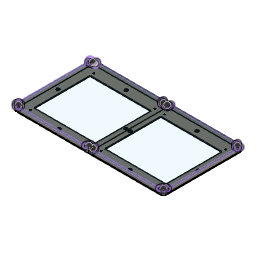
v1.1 (Autodesk Fusion 360 design; units mm, degrees)
Autodesk Fusion 360 part; units mm, degrees
sketch "Sketch1" plane through (0, 0, 0) normal (0, 0, 1) x (1, 0, 0)
  line L0 (192.1478, -6) -> (205.1478, -6) construction
  line L1 (192.1478, -6) -> (179.1478, -6) construction
  circle A0 centre (179.1461, -187.9671) radius 2
  circle A1 centre (13.1478, -188) radius 2
  line L2 (13.1478, -6) -> (13.1478, -16) construction
  circle A2 centre (205.1478, -16) radius 2
  line L3 (13.1478, -198) -> (13.1478, -188) construction
  line L4 (384.1478, -198) -> (371.1478, -198) construction
  line L5 (179.1478, -26) -> (13.1478, -26)
  line L6 (192.1478, -197.9671) -> (179.1478, -197.9671) construction
  line L7 (384.1478, -6) -> (371.1478, -6) construction
  line L8 (179.1478, -6) -> (179.1478, -26) construction
  line L9 (192.1478, -197.9671) -> (0.1478, -198)
  line L10 (205.1478, -197.9671) -> (205.1478, -187.9671) construction
  line L11 (0.1478, -198) -> (0.1478, -6)
  circle A3 centre (179.1478, -16) radius 2
  line L12 (384.1478, -198) -> (384.1478, -6)
  line L13 (371.1478, -26) -> (205.1478, -26)
  line L14 (371.1478, -198) -> (371.1478, -188) construction
  line L15 (205.1478, -26) -> (205.1478, -177.9671)
  line L16 (13.1478, -178) -> (179.1478, -178)
  line L17 (0.1478, -198) -> (13.1478, -198) construction
  line L18 (205.1478, -197.9671) -> (205.1478, -177.9671) construction
  circle A4 centre (205.1478, -187.9671) radius 2
  line L19 (0.1478, -198) -> (13.1478, -198) construction
  line L20 (371.1478, -6) -> (371.1478, -16) construction
  line L21 (192.1478, -6) -> (179.1478, -6) construction
  circle A5 centre (13.1478, -16) radius 2
  circle A6 centre (371.1478, -16) radius 2
  line L22 (192.1478, -6) -> (192.1478, -197.9671) construction
  line L23 (179.1478, -6) -> (179.1478, -16) construction
  line L24 (371.1478, -6) -> (371.1478, -26) construction
  line L25 (205.1478, -6) -> (205.1478, -16) construction
  line L26 (13.1478, -26) -> (13.1478, -178)
  line L27 (384.1478, -6) -> (0.1478, -6)
  line L28 (179.1478, -197.9671) -> (179.1461, -187.9671) construction
  line L29 (13.1478, -198) -> (13.1478, -178) construction
  line L30 (0.1478, -6) -> (13.1478, -6) construction
  line L31 (179.1478, -178) -> (179.1478, -26)
  line L32 (192.1478, -197.9671) -> (205.1478, -197.9671) construction
  line L33 (0.1478, -6) -> (0.1478, -198)
  line L34 (205.1478, -177.9671) -> (371.1478, -177.9671)
  circle A7 centre (371.1478, -188) radius 2
  line L35 (384.1478, -6) -> (371.1478, -6) construction
  line L36 (371.1478, -177.9671) -> (371.1478, -26)
  line L37 (0.1478, -198) -> (384.1478, -198)
  line L38 (192.1478, -197.9671) -> (205.1478, -197.9671) construction
  line L39 (384.1478, -6) -> (384.1478, 12.0213) construction
  line L40 (0.1478, -6) -> (-9.0446, 3.1924) construction
  line L41 (0.1478, -6) -> (15, -6) construction
  circle A8 centre (-4.4484, -1.4038) radius 6.5
  line L42 (0.1478, -198) -> (-9.0446, -207.1924) construction
  line L43 (384.1478, -198) -> (393.3402, -207.1924) construction
  line L44 (384.1478, -198) -> (399, -198) construction
  line L45 (384.1478, -6) -> (393.3402, 3.1924) construction
  line L46 (384.1478, -6) -> (399, -6) construction
  circle A9 centre (388.744, -1.4038) radius 6.5
  circle A10 centre (388.744, -202.5962) radius 6.5
  circle A11 centre (-4.4484, -202.5962) radius 6.5
  line L47 (-10.9305, -1.8855) -> (-10.9484, -202.5956)
  line L48 (-4.4484, -209.0962) -> (388.744, -209.0962)
  line L49 (395.244, -202.5962) -> (395.244, -1.4038)
  line L50 (-4.4484, 5.0962) -> (388.744, 5.0962)
  line L51 (388.744, -202.5962) -> (395.244, -202.5962) construction
  line L52 (-4.4484, -1.4038) -> (-4.4484, 5.0962) construction
  point P0 (13, -13)
  dimension "d13" = 192
  dimension "d14" = 192
  dimension "d15" = 384
  dimension "d16" = 384
  dimension "d20" = 13
  dimension "d21" = 10
  dimension "d22" = 4
  dimension "d23" = 13
  dimension "d24" = 10
  dimension "d25" = 13
  dimension "d26" = 10
  dimension "d27" = 13
  dimension "d28" = 10
  dimension "d29" = 13
  dimension "d30" = 10
  dimension "d31" = 13
  dimension "d32" = 10
  dimension "d33" = 13
  dimension "d34" = 10
  dimension "d35" = 13
  dimension "d36" = 10
  dimension "d37" = 4
  dimension "d38" = 4
  dimension "d39" = 4
  dimension "d40" = 4
  dimension "d41" = 4
  dimension "d42" = 4
  dimension "d43" = 4
  dimension "d44" = 13
  dimension "d45" = 20
  dimension "d46" = 13
  dimension "d47" = 20
  dimension "d48" = 13
  dimension "d49" = 20
  dimension "d50" = 13
  dimension "d51" = 20
  dimension "d69" = 135
  dimension "d70" = 13
  dimension "d71" = 13
  dimension "d72" = 45
  dimension "d73" = 13
  dimension "d74" = 13
  dimension "d75" = 45
  dimension "d104" = 135
  constraint perpendicular L11 L30
  constraint perpendicular L2 L30
  constraint coincident L2.end A5.centre
  constraint perpendicular L7 L12
  constraint perpendicular L7 L20
  constraint perpendicular L4 L12
  constraint perpendicular L14 L37
  constraint perpendicular L19 L33
  constraint perpendicular L3 L19
  constraint midpoint L0.start L27
  constraint perpendicular L22 L37
  constraint perpendicular L6 L22
  constraint perpendicular L9 L28
  constraint perpendicular L21 L22
  constraint perpendicular L21 L23
  constraint perpendicular L0 L22
  constraint perpendicular L25 L27
  constraint perpendicular L22 L32
  constraint perpendicular L10 L32
  constraint coincident A1.centre L3.end
  constraint coincident A3.centre L23.end
  constraint coincident A0.centre L28.end
  constraint coincident A2.centre L25.end
  constraint coincident L10.end A4.centre
  constraint coincident L14.end A7.centre
  constraint coincident L20.end A6.centre
  constraint perpendicular L11 L17
  constraint perpendicular L17 L29
  constraint perpendicular L1 L22
  constraint perpendicular L1 L8
  constraint horizontal L16
  constraint vertical L31
  constraint horizontal L5
  constraint vertical L26
  constraint perpendicular L22 L38
  constraint perpendicular L18 L38
  constraint perpendicular L20 L35
  constraint perpendicular L24 L35
  constraint horizontal L34
  constraint vertical L36
  constraint horizontal L13
  constraint vertical L15
  constraint perpendicular L7 L39
  constraint horizontal L41
  constraint coincident L40.end A8
  constraint coincident L11.end A8
  constraint horizontal L44
  constraint horizontal L46
  constraint coincident L45.end A9
  constraint coincident L7.start A9
  constraint coincident L43.end A10
  constraint coincident L4.start A10
  constraint coincident L42.end A11
  constraint coincident L9.end A11
  constraint coincident A8 L47.start
  constraint coincident A11 L47.end
  constraint tangent A11 L47
  constraint coincident A10 L48.end
  constraint tangent A10 L48
  constraint coincident A9 L49.end
  constraint tangent A9 L49
  constraint perpendicular L46 L49
  constraint coincident A9 L50.end
  constraint tangent A9 L50
  constraint perpendicular L49 L50
  constraint coincident L42 A11.centre
  constraint coincident L43 A10.centre
  constraint coincident L45 A9.centre
  constraint coincident L40 A8.centre
  constraint coincident A11 L48.start
  constraint tangent A11 L48
  constraint coincident A10.centre L51.start
  constraint coincident A10 L49.start
  constraint parallel L48 L51
  constraint coincident L49.start L51.end
  constraint coincident A8.centre L52.start
  constraint coincident A8 L50.start
  constraint vertical L52
  constraint coincident L50.start L52.end
  measures "d13" distance of L11.end L9.end
  measures "d14" distance of L4.start L7.start
  measures "d15" distance of L7.start L11.end
  measures "d16" distance of L4.start L9.end
  measures "d20" distance of L2.start L11.end
  measures "d21" distance of L2.start L2.end
  measures "d22" diameter of A5
  measures "d23" distance of L7.end L7.start
  measures "d24" distance of L7.end L20.end
  measures "d25" distance of L4.end L4.start
  measures "d26" distance of L4.end L14.end
  measures "d27" distance of L3.start L9.end
  measures "d28" distance of L3.start A1.centre
  measures "d29" distance of L6.end L6.start
  measures "d30" distance of L6.end A0.centre
  measures "d31" distance of L0.start L1.end
  measures "d32" distance of A3.centre L1.end
  measures "d33" distance of L0.start L0.end
  measures "d34" distance of A2.centre L0.end
  measures "d35" distance of L10.start L6.start
  measures "d36" distance of L10.end L10.start
  measures "d37" diameter of A1
  measures "d38" diameter of A3
  measures "d39" diameter of A0
  measures "d40" diameter of A2
  measures "d41" diameter of A4
  measures "d42" diameter of A7
  measures "d43" diameter of A6
  measures "d44" distance of L9.end L3.start
  measures "d45" distance of L16.start L3.start
  measures "d46" distance of L0.start L1.end
  measures "d47" distance of L5.start L1.end
  measures "d48" distance of L6.start L10.start
  measures "d49" distance of L10.start L15.end
  measures "d50" distance of L7.start L7.end
  measures "d51" distance of L13.start L7.end
  measures "d69" angle of L40 L41
  measures "d70" distance of L11.end L40.end
  measures "d71" distance of L9.end L42.end
  measures "d72" angle of L43 L44
  measures "d73" distance of L4.start L43.end
  measures "d74" distance of L7.start L45.end
  measures "d75" angle of L45 L46
  measures "d104" angle of L37 L42
extrude "Extrude1" add sketch "Sketch1" along normal blind 2 makes body 1
sketch "Sketch3" plane through (0, 0, 2) normal (0, 0, 1) x (-1, 0, 0)
  arc A0 (-395.244, 1.4038) -> (-388.744, -5.0962) centre (-388.744, 1.4038) ccw
  line L0 (-388.744, -5.0962) -> (4.4484, -5.0962)
  arc A1 (4.4484, -5.0962) -> (10.9305, 1.8855) centre (4.4484, 1.4038) ccw
  circle A2 centre (4.4484, 1.4038) radius 5.5
  circle A3 centre (4.4484, 202.5962) radius 5.5
  circle A4 centre (-388.744, 202.5962) radius 5.5
  circle A5 centre (-388.744, 1.4038) radius 5.5
  line L1 (-388.744, -4.0962) -> (4.4484, -4.0962)
  line L2 (9.9484, 1.4038) -> (9.9484, 202.5962)
  line L3 (3.3138, 207.9779) -> (-388.7423, 208.0962)
  line L4 (-394.244, 202.5962) -> (-394.244, 1.4038)
  line L5 (-192.1478, -4.0962) -> (-192.7143, 208.037) construction
  circle A6 centre (-187.1611, 0.9038) radius 5
  circle A7 centre (-197.1612, 0.9038) radius 5
  circle A8 centre (-187.7009, 203.0355) radius 5
  circle A9 centre (-197.701, 203.0385) radius 5
  line L6 (-182.7009, 203.0355) -> (-182.7009, 208.034)
  line L7 (-202.7008, 203.0726) -> (-202.667, 208.04)
  line L8 (-187.1611, 5.9038) -> (-197.1612, 5.9038)
  line L9 (-202.1612, 0.9038) -> (-202.1612, -4.0962)
  line L10 (-182.1611, 0.9038) -> (-182.1611, -4.0962)
  line L11 (-383.662, 197.9997) -> (-384, 6)
  line L12 (0.338, 197.9997) -> (-383.662, 197.9997)
  line L13 (0, 6) -> (0.338, 197.9997)
  line L14 (-384, 6) -> (0, 6)
  line L15 (4.4484, 6.9038) -> (9.9484, 6.9038)
  line L16 (-1.0516, 1.4038) -> (-1.0516, -4.0962)
  line L17 (-383.244, 1.4038) -> (-383.244, -4.0962)
  line L18 (-388.744, 6.9038) -> (-394.244, 6.9038)
  line L19 (-388.744, 197.0962) -> (-394.244, 197.0962)
  line L20 (-383.244, 202.5962) -> (-383.244, 208.0945)
  line L21 (4.4484, 197.0962) -> (9.9484, 197.0962)
  line L22 (-1.0516, 202.5962) -> (-1.0516, 207.9792)
  circle A10 centre (-13.1478, 188) radius 2
  circle A11 centre (-179.1461, 187.9671) radius 2
  circle A12 centre (-205.1478, 16) radius 2
  circle A13 centre (-179.1478, 16) radius 2
  circle A14 centre (-205.1478, 187.9671) radius 2
  circle A15 centre (-13.1478, 16) radius 2
  circle A16 centre (-371.1478, 16) radius 2
  line L23 (-179.1478, 26) -> (-179.1478, 178)
  line L24 (-179.1478, 178) -> (-13.1478, 178)
  line L25 (-13.1478, 178) -> (-13.1478, 26)
  line L26 (-13.1478, 26) -> (-179.1478, 26)
  line L27 (-371.1478, 26) -> (-371.1478, 177.9671)
  line L28 (-371.1478, 177.9671) -> (-205.1478, 177.9671)
  line L29 (-205.1478, 177.9671) -> (-205.1478, 26)
  line L30 (-205.1478, 26) -> (-371.1478, 26)
  circle A17 centre (-371.1478, 188) radius 2
  line L31 (10.9305, 1.8855) -> (10.9484, 202.5956)
  arc A18 (10.9484, 202.5956) -> (4.4484, 209.0962) centre (4.4484, 202.5962) ccw
  line L32 (4.4484, 209.0962) -> (-388.744, 209.0962)
  arc A19 (-388.744, 209.0962) -> (-395.244, 202.5962) centre (-388.744, 202.5962) ccw
  line L33 (-395.244, 202.5962) -> (-395.244, 1.4038)
  line L34 (-187.7009, 198.0355) -> (-197.7025, 198.0385)
  dimension "d76" = 11
  dimension "d77" = 11
  dimension "d78" = 11
  dimension "d79" = 11
  dimension "d80" = 5
  dimension "d81" = 5
  dimension "d82" = 5
  dimension "d83" = 5
  dimension "d85" = 192
  dimension "d87" = 384
  constraint concentric A1 A2
  constraint concentric A0 A5
  constraint coincident A5 L1.start
  constraint coincident A2 L1.end
  constraint tangent A2 L1
  constraint parallel L0 L1
  constraint coincident A2 L2.start
  constraint coincident A3 L2.end
  constraint tangent A3 L2
  constraint coincident A3 L3.start
  constraint coincident A4 L3.end
  constraint tangent A4 L3
  constraint coincident A4 L4.start
  constraint coincident A5 L4.end
  constraint tangent A5 L4
  constraint midpoint L1 L5.start
  constraint midpoint L3 L5.end
  constraint tangent L1 A6
  constraint tangent L5 A6
  constraint tangent L5 A7
  constraint tangent L1 A7
  constraint tangent L5 A8
  constraint tangent L3 A8
  constraint tangent L5 A9
  constraint tangent L3 A9
  constraint coincident A8 L6.start
  constraint coincident L3 L6.end
  constraint tangent A8 L6
  constraint vertical L6
  constraint coincident A9 L7.start
  constraint coincident L3 L7.end
  constraint tangent A9 L7
  constraint coincident A6 L8.start
  constraint coincident A7 L8.end
  constraint tangent A7 L8
  constraint horizontal L8
  constraint coincident A7 L9.start
  constraint coincident L1 L9.end
  constraint tangent A7 L9
  constraint perpendicular L1 L9
  constraint coincident A6 L10.start
  constraint coincident L1 L10.end
  constraint tangent A6 L10
  constraint perpendicular L1 L10
  constraint coincident A2 L15.start
  constraint coincident L2 L15.end
  constraint tangent A2 L15
  constraint horizontal L15
  constraint coincident A2 L16.start
  constraint coincident L1 L16.end
  constraint tangent A2 L16
  constraint perpendicular L1 L16
  constraint coincident A5 L17.start
  constraint coincident L1 L17.end
  constraint tangent A5 L17
  constraint perpendicular L1 L17
  constraint coincident A5 L18.start
  constraint coincident L4 L18.end
  constraint tangent A5 L18
  constraint perpendicular L4 L18
  constraint coincident A4 L19.start
  constraint coincident L4 L19.end
  constraint tangent A4 L19
  constraint perpendicular L4 L19
  constraint coincident A4 L20.start
  constraint coincident L3 L20.end
  constraint tangent A4 L20
  constraint vertical L20
  constraint coincident A3 L21.start
  constraint coincident L2 L21.end
  constraint tangent A3 L21
  constraint horizontal L21
  constraint coincident A3 L22.start
  constraint coincident L3 L22.end
  constraint tangent A3 L22
  constraint vertical L22
  constraint coincident A3.centre A18.centre
  constraint coincident A4.centre A19.centre
  constraint coincident A8 L34.start
  constraint coincident A9 L34.end
  constraint tangent A9 L34
  measures "d76" diameter of A2
  measures "d77" diameter of A3
  measures "d78" diameter of A4
  measures "d79" diameter of A5
  measures "d80" radius of A6
  measures "d81" radius of A7
  measures "d82" radius of A8
  measures "d83" radius of A9
  measures "d85" distance of L13.start L12.start
  measures "d87" distance of L13.start L11.end
extrude "Extrude3" add sketch "Sketch3" along normal blind 10.5 contours A0 L0 A1 L31 A18 L32 A19 L33 | A2 | A2 L2 L15 | A8 A9 L34 | A2 L1 L16 | A3 L2 L21 | L1 A6 L10 | A3 | L1 A6 A7 | A6 | A3 L3 L22 | L1 A7 L9 | A7 | A6 A7 L8 | L3 A8 L6 | A5 L1 L17 | L3 A8 A9 | A8 | A5 | L3 A9 L7 | A9 | A5 L4 L18 | A4 L3 L20 | A4 L4 L19 | A4 bodies 1
sketch "Sketch4" plane through (0, 0, 12.5) normal (0, 0, 1) x (-1, 0, 0)
  arc A0 (4.4484, -5.0962) -> (10.9305, 1.8855) centre (4.4484, 1.4038) ccw
  line L0 (-388.744, -5.0962) -> (4.4484, -5.0962)
  circle A1 centre (4.4484, 1.4038) radius 5
  circle A2 centre (-187.1611, 0.9038) radius 5
  circle A3 centre (-197.1612, 0.9038) radius 5
  circle A4 centre (-388.744, 1.4038) radius 5
  circle A5 centre (-388.744, 202.5962) radius 5
  circle A6 centre (-197.701, 203.0385) radius 5
  circle A7 centre (-187.7009, 203.0355) radius 5
  circle A8 centre (4.4484, 202.5962) radius 5
  line L1 (10.9305, 1.8855) -> (10.9484, 202.5956)
  arc A9 (10.9484, 202.5956) -> (4.4484, 209.0962) centre (4.4484, 202.5962) ccw
  line L2 (4.4484, 209.0962) -> (-388.744, 209.0962)
  arc A10 (-388.744, 209.0962) -> (-395.244, 202.5962) centre (-388.744, 202.5962) ccw
  line L3 (-395.244, 202.5962) -> (-395.244, 1.4038)
  arc A11 (-395.244, 1.4038) -> (-388.744, -5.0962) centre (-388.744, 1.4038) ccw
  line L4 (-202.1612, -4.0962) -> (-383.244, -4.0962)
  arc A12 (-383.244, 1.4038) -> (-388.744, 6.9038) centre (-388.744, 1.4038) ccw
  line L5 (-394.244, 6.9038) -> (-394.244, 197.0962)
  arc A13 (-388.744, 197.0962) -> (-383.244, 202.5962) centre (-388.744, 202.5962) ccw
  line L6 (-383.244, 208.0945) -> (-202.667, 208.04)
  arc A14 (-1.0516, 202.5962) -> (4.4484, 197.0962) centre (4.4484, 202.5962) ccw
  line L7 (9.9484, 197.0962) -> (9.9484, 6.9038)
  arc A15 (4.4484, 6.9038) -> (-1.0516, 1.4038) centre (4.4484, 1.4038) ccw
  arc A16 (-187.7009, 198.0355) -> (-182.7009, 203.0355) centre (-187.7009, 203.0355) ccw
  line L8 (-182.7009, 203.0355) -> (-182.7009, 208.034)
  line L9 (-182.7009, 208.034) -> (-1.0516, 207.9792)
  line L10 (-1.0516, 207.9792) -> (-1.0516, 202.5962)
  line L11 (4.4484, 197.0962) -> (9.9484, 197.0962)
  line L12 (9.9484, 6.9038) -> (4.4484, 6.9038)
  line L13 (-1.0516, 1.4038) -> (-1.0516, -4.0962)
  line L14 (-1.0516, -4.0962) -> (-182.1611, -4.0962)
  line L15 (-182.1611, -4.0962) -> (-182.1611, 0.9038)
  arc A17 (-182.1611, 0.9038) -> (-187.1611, 5.9038) centre (-187.1611, 0.9038) ccw
  line L16 (-187.1611, 5.9038) -> (-197.1612, 5.9038)
  arc A18 (-197.1612, 5.9038) -> (-202.1612, 0.9038) centre (-197.1612, 0.9038) ccw
  line L17 (-202.1612, 0.9038) -> (-202.1612, -4.0962)
  line L18 (-394.244, 197.0962) -> (-388.744, 197.0962)
  line L19 (-383.244, 202.5962) -> (-383.244, 208.0945)
  line L20 (-202.667, 208.04) -> (-202.7008, 203.0726)
  arc A19 (-202.7008, 203.0726) -> (-197.7025, 198.0385) centre (-197.701, 203.0385) ccw
  line L21 (-197.7025, 198.0385) -> (-187.7009, 198.0355)
  line L22 (-383.244, -4.0962) -> (-383.244, 1.4038)
  line L23 (-388.744, 6.9038) -> (-394.244, 6.9038)
  point P0 (3.9781, 2.1111)
  dimension "d90" = 10
  dimension "d91" = 10
  dimension "d92" = 10
  dimension "d93" = 10
  dimension "d94" = 10
  dimension "d95" = 10
  dimension "d96" = 10
  dimension "d97" = 10
  constraint coincident A2.centre A17.centre
  constraint coincident A3.centre A18.centre
  constraint coincident A5.centre A10.centre
  constraint coincident A4.centre A11.centre
  constraint coincident A6.centre A19.centre
  constraint coincident A7.centre A16.centre
  constraint coincident A8.centre A9.centre
  constraint coincident A0.centre A1.centre
  measures "d90" diameter of A1
  measures "d91" diameter of A2
  measures "d92" diameter of A3
  measures "d93" diameter of A4
  measures "d94" diameter of A5
  measures "d95" diameter of A6
  measures "d96" diameter of A7
  measures "d97" diameter of A8
extrude "Extrude4" cut sketch "Sketch4" against normal blind 3.2 contours A1 | A2 A17 | A3 A18 | A7 A16 | A6 A19 | A4 | A5 | A8 bodies 1
extrude "Extrude5" add 3 faces at (-9.9182, -4.1722, 12.5) (192.3118, -3.3983, 12.5) (192.5511, -200.5431, 12.5) along direction (0, 0, 1) blind 3 separate body on bodies 1 makes body 2
sketch "Sketch7" plane through (0, 0, 15.5) normal (0, 0, 1) x (-1, 0, 0)
  arc A0 (-197.7025, 198.0385) -> (-202.7008, 203.0726) centre (-197.701, 203.0385) ccw
  line L0 (-197.7025, 198.0385) -> (-187.7009, 198.0355)
  arc A1 (-182.7009, 203.0355) -> (-187.7009, 198.0355) centre (-187.7009, 203.0355) ccw
  line L1 (-182.7009, 203.0355) -> (-182.7009, 208.034)
  line L2 (-182.7009, 208.034) -> (-1.0516, 207.9792)
  line L3 (-1.0516, 207.9792) -> (-1.0516, 202.5962)
  arc A2 (-1.0516, 202.5962) -> (4.4484, 197.0962) centre (4.4484, 202.5962) ccw
  line L4 (4.4484, 197.0962) -> (9.9484, 197.0962)
  line L5 (9.9484, 197.0962) -> (9.9484, 6.9038)
  line L6 (9.9484, 6.9038) -> (4.4484, 6.9038)
  arc A3 (4.4484, 6.9038) -> (-1.0516, 1.4038) centre (4.4484, 1.4038) ccw
  line L7 (-1.0516, 1.4038) -> (-1.0516, -4.0962)
  line L8 (-1.0516, -4.0962) -> (-182.1611, -4.0962)
  line L9 (-182.1611, -4.0962) -> (-182.1611, 0.9038)
  arc A4 (-187.1611, 5.9038) -> (-182.1611, 0.9038) centre (-187.1611, 0.9038) ccw
  line L10 (-187.1611, 5.9038) -> (-197.1612, 5.9038)
  arc A5 (-202.1612, 0.9038) -> (-197.1612, 5.9038) centre (-197.1612, 0.9038) ccw
  line L11 (-202.1612, 0.9038) -> (-202.1612, -4.0962)
  line L12 (-202.1612, -4.0962) -> (-383.244, -4.0962)
  line L13 (-383.244, -4.0962) -> (-383.244, 1.4038)
  arc A6 (-383.244, 1.4038) -> (-388.744, 6.9038) centre (-388.744, 1.4038) ccw
  line L14 (-388.744, 6.9038) -> (-394.244, 6.9038)
  line L15 (-394.244, 6.9038) -> (-394.244, 197.0962)
  line L16 (-394.244, 197.0962) -> (-388.744, 197.0962)
  arc A7 (-388.744, 197.0962) -> (-383.244, 202.5962) centre (-388.744, 202.5962) ccw
  line L17 (-383.244, 202.5962) -> (-383.244, 208.0945)
  line L18 (-383.244, 208.0945) -> (-202.667, 208.04)
  line L19 (-202.667, 208.04) -> (-202.7008, 203.0726)
  circle A8 centre (-388.744, 202.5962) radius 5
  circle A9 centre (4.4484, 1.4038) radius 5
  circle A10 centre (-388.744, 1.4038) radius 5
  circle A11 centre (4.4484, 202.5962) radius 5
  line L20 (-395.244, 202.5962) -> (-395.244, 1.4038)
  arc A12 (-395.244, 1.4038) -> (-388.744, -5.0962) centre (-388.744, 1.4038) ccw
  line L21 (-388.744, -5.0962) -> (4.4484, -5.0962)
  arc A13 (4.4484, -5.0962) -> (10.9305, 1.8855) centre (4.4484, 1.4038) ccw
  line L22 (10.9305, 1.8855) -> (10.9484, 202.5956)
  arc A14 (10.9484, 202.5956) -> (4.4484, 209.0962) centre (4.4484, 202.5962) ccw
  line L23 (4.4484, 209.0962) -> (-388.744, 209.0962)
  arc A15 (-388.744, 209.0962) -> (-395.244, 202.5962) centre (-388.744, 202.5962) ccw
  circle A16 centre (4.4484, 202.5962) radius 6.5
  circle A17 centre (4.4484, 1.4038) radius 6.5
  circle A18 centre (-388.744, 1.4038) radius 6.5
  circle A19 centre (-388.744, 202.5962) radius 6.5
  spline S0 degree 5 poles (10.9467, 1.2553) (10.9468, 9.309) (10.9469, 25.4162) (10.9471, 49.577) (10.9474, 81.7915) (10.9477, 122.0595) (10.948, 154.274) (10.9482, 178.4348) (10.9483, 194.542) (10.9484, 202.5956) knots 0 0 0 0 0 0 0.2 0.4 0.6 0.8 1 1 1 1 1 1
  line L24 (4.4484, 209.0962) -> (-388.744, 209.0962)
  line L25 (-395.244, 202.5962) -> (-395.244, 1.4038)
  line L26 (-388.744, -5.0962) -> (4.4484, -5.0962)
  constraint concentric A2 A16
  constraint concentric A3 A17
  constraint concentric A6 A18
  constraint concentric A7 A19
  constraint coincident A13 S0.start
  constraint coincident A17 S0.start
  constraint coincident L22.end A14.start
  constraint coincident A14.end L23.start
  constraint coincident L23.end A15.start
  constraint coincident L20.start A15.end
  constraint coincident L20.end A12.start
  constraint coincident A12.end L21.start
  constraint coincident L21.end A13.start
extrude "Extrude7" add sketch "Sketch7" along normal blind 0.5 contours A4 L10 A5 | A0 A1 L1 L2 L3 L4 L5 L6 L7 L8 L9 A4 A5 L11 L12 L13 L14 L15 L16 L17 L18 L19 A16 A17 A18 A19 | A0 A1 L1 L2 L3 L17 L18 L19 L23 A16 A19 L24 | A0 L0 A1 | L16 A7 L17 A19 | L16 A7 L17 A15 A19 | L3 A2 L4 A14 A16 | L3 A2 L4 A16 | L4 L5 L6 L22 A16 A17 S0 | L14 L15 L16 L20 A18 A19 L25 | L13 A6 L14 A12 A18 | L6 A3 L7 A13 A17 S0 | L7 L8 L9 A4 A5 L11 L12 L13 L21 A17 A18 L26 | L13 A6 L14 A18 | L6 A3 L7 A17 | A8 | A9 | A10 | A11 bodies 2
sketch "Sketch8" plane through (0, 0, 2) normal (0, 0, 1) x (-1, 0, 0)
  line L0 (-197.1612, 5.9038) -> (-187.1611, 5.9038)
  arc A0 (-182.1611, 0.9038) -> (-187.1611, 5.9038) centre (-187.1611, 0.9038) ccw
  line L1 (-182.1611, 0.9038) -> (-182.1611, -4.0962)
  line L2 (-182.1611, -4.0962) -> (-1.0516, -4.0962)
  line L3 (-1.0516, -4.0962) -> (-1.0516, 1.4038)
  arc A1 (4.4484, 6.9038) -> (-1.0516, 1.4038) centre (4.4484, 1.4038) ccw
  line L4 (4.4484, 6.9038) -> (9.9484, 6.9038)
  line L5 (9.9484, 6.9038) -> (9.9484, 197.0962)
  line L6 (9.9484, 197.0962) -> (4.4484, 197.0962)
  arc A2 (-1.0516, 202.5962) -> (4.4484, 197.0962) centre (4.4484, 202.5962) ccw
  line L7 (-1.0516, 202.5962) -> (-1.0516, 207.9792)
  line L8 (-1.0516, 207.9792) -> (-182.7009, 208.034)
  line L9 (-182.7009, 208.034) -> (-182.7009, 203.0355)
  arc A3 (-187.7009, 198.0355) -> (-182.7009, 203.0355) centre (-187.7009, 203.0355) ccw
  line L10 (-187.7009, 198.0355) -> (-197.7025, 198.0385)
  circle A4 centre (-179.1478, 16) radius 2
  circle A5 centre (-13.1478, 16) radius 2
  line L11 (-179.1478, 26) -> (-179.1478, 178)
  line L12 (-179.1478, 178) -> (-13.1478, 178)
  line L13 (-13.1478, 178) -> (-13.1478, 26)
  line L14 (-13.1478, 26) -> (-179.1478, 26)
  circle A6 centre (-13.1478, 188) radius 2
  circle A7 centre (-179.1461, 187.9671) radius 2
  line L15 (-13.1478, 102) -> (-179.1478, 102) construction
  line L16 (-96.1478, 26) -> (-96.1478, 178) construction
  line L17 (-96.1478, 26) -> (-96.1478, -4.0962) construction
  line L18 (-13.1478, 102) -> (9.9484, 102) construction
  line L19 (-179.1478, 102) -> (-179.1526, 101.9998) construction
  line L20 (-179.1526, 101.9998) -> (-194.2518, 101.9998) construction
  line L21 (-96.1478, 178) -> (-96.1388, 208.0079) construction
  circle A8 centre (-96.1478, 10.9519) radius 4
  circle A9 centre (-1.5997, 102) radius 4
  circle A10 centre (-186.7022, 101.9998) radius 4
  circle A11 centre (-96.1433, 193.004) radius 4
  circle A12 centre (-288.1649, 10.9605) radius 4
  circle A13 centre (-382.7049, 102.017) radius 4
  circle A14 centre (-288.1532, 193.0125) radius 4
  circle A15 centre (-198.2326, 101.9709) radius 4
  line L22 (-194.2963, 43.9518) -> (-190.2963, 43.9518)
  line L23 (-190.2963, 43.9518) -> (-190.2963, 63.9518)
  line L24 (-190.2963, 63.9518) -> (-194.2963, 63.9518)
  line L25 (-194.2963, 63.9518) -> (-194.2963, 43.9518)
  line L26 (-194.2963, 43.9518) -> (-190.2963, 63.9518) construction
  line L27 (-190.2963, 43.9518) -> (-194.2963, 63.9518) construction
  line L28 (-190.5666, 160.0184) -> (-194.5666, 160.0184)
  line L29 (-194.5666, 160.0184) -> (-194.5666, 140.0184)
  line L30 (-194.5666, 140.0184) -> (-190.5666, 140.0184)
  line L31 (-190.5666, 140.0184) -> (-190.5666, 160.0184)
  line L32 (-190.5666, 160.0184) -> (-194.5666, 140.0184) construction
  line L33 (-194.5666, 160.0184) -> (-190.5666, 140.0184) construction
  arc A16 (-202.7008, 203.0726) -> (-197.7025, 198.0385) centre (-197.701, 203.0385) ccw
  line L34 (-202.7008, 203.0726) -> (-202.667, 208.04)
  line L35 (-202.667, 208.04) -> (-383.244, 208.0945)
  line L36 (-383.244, 208.0945) -> (-383.244, 202.5962)
  arc A17 (-388.744, 197.0962) -> (-383.244, 202.5962) centre (-388.744, 202.5962) ccw
  line L37 (-388.744, 197.0962) -> (-394.244, 197.0962)
  line L38 (-394.244, 197.0962) -> (-394.244, 6.9038)
  line L39 (-394.244, 6.9038) -> (-388.744, 6.9038)
  arc A18 (-383.244, 1.4038) -> (-388.744, 6.9038) centre (-388.744, 1.4038) ccw
  line L40 (-383.244, 1.4038) -> (-383.244, -4.0962)
  line L41 (-383.244, -4.0962) -> (-202.1612, -4.0962)
  line L42 (-202.1612, -4.0962) -> (-202.1612, 0.9038)
  arc A19 (-197.1612, 5.9038) -> (-202.1612, 0.9038) centre (-197.1612, 0.9038) ccw
  circle A20 centre (-205.1478, 16) radius 2
  circle A21 centre (-205.1478, 187.9671) radius 2
  circle A22 centre (-371.1478, 16) radius 2
  line L43 (-371.1478, 26) -> (-371.1478, 177.9671)
  line L44 (-371.1478, 177.9671) -> (-205.1478, 177.9671)
  line L45 (-205.1478, 177.9671) -> (-205.1478, 26)
  line L46 (-205.1478, 26) -> (-371.1478, 26)
  circle A23 centre (-371.1478, 188) radius 2
  line L47 (-192.7017, 198.037) -> (-192.4315, 101.9998) construction
  line L48 (-192.4315, 101.9998) -> (-192.1612, 5.9038) construction
  line L49 (-179.1526, 101.9998) -> (-190.7022, 101.9926)
  line L50 (-192.4315, 101.9915) -> (-205.1478, 101.9836)
  line L51 (-190.7022, 101.9926) -> (-192.4315, 101.9915)
  point P0 (-192.2963, 53.9518)
  point P1 (-192.5666, 150.0184)
  dimension "d107" = 8
  dimension "d108" = 8
  dimension "d109" = 8
  dimension "d110" = 8
  dimension "d119" = 4
  dimension "d120" = 20
  dimension "d121" = 4
  dimension "d122" = 20
  constraint midpoint L13 L15.start
  constraint midpoint L11 L15.end
  constraint midpoint L14 L16.start
  constraint midpoint L12 L16.end
  constraint coincident L2 L17.end
  constraint perpendicular L2 L17
  constraint midpoint L5 L18.end
  constraint horizontal L20
  constraint coincident L8 L21.end
  constraint perpendicular L8 L21
  constraint midpoint L17 A8.centre
  constraint midpoint L18 A9.centre
  constraint midpoint L20 A10.centre
  constraint midpoint L21 A11.centre
  constraint horizontal L22
  constraint perpendicular L22 L23
  constraint parallel L22 L24
  constraint parallel L23 L25
  constraint coincident L26 P0
  constraint coincident L27 P0
  constraint horizontal L28
  constraint perpendicular L28 L29
  constraint parallel L28 L30
  constraint parallel L29 L31
  constraint coincident L32 P1
  constraint coincident L33 P1
  constraint midpoint L10 L47.start
  constraint midpoint L0 L48.end
  constraint coincident L20 L47.end
  constraint midpoint P0 L48
  constraint midpoint P1 L47
  constraint midpoint L45 L50.end
  constraint coincident A10 L49.end
  constraint coincident L48 L50.start
  measures "d107" diameter of A8
  measures "d108" diameter of A9
  measures "d109" diameter of A10
  measures "d110" diameter of A11
  measures "d119" distance of L23.end L24.end
  measures "d120" distance of L22.end L23.end
  measures "d121" distance of L29.end L30.end
  measures "d122" distance of L28.end L29.end
extrude "Extrude8" cut sketch "Sketch8" against normal blind 1 contours A8 | A9 | A10 L49 | A10 L49 | A11 | A12 | A13 | A14 | A15 L50 | A15 L50 bodies 1
ref_plane "WorkPlane3" through (192.1523, -102.2541, 6.25) normal (-1, 0.000045, 0) x (-0.000045, -1, 0)
sketch "Sketch9" plane through (0, 0, 1) normal (0, 0, 1) x (-1, 0, 0)
  circle A0 centre (-96.1478, 10.9519) radius 4
  circle A1 centre (-96.1478, 10.9519) radius 2
  circle A2 centre (-96.15, 193) radius 4.0003 construction
  circle A3 centre (-186.0715, 101.9648) radius 3.9976 construction
  circle A4 centre (-1.5965, 102.0007) radius 3.9975 construction
  circle A5 centre (-1.5965, 102.0007) radius 2
  circle A6 centre (-96.15, 193) radius 2
  circle A7 centre (-186.0715, 101.9648) radius 2
  line L0 (-192.1469, 222.691) -> (-192.1576, -18.4505)
  circle A8 centre (-382.7081, 102.0177) radius 2
  circle A9 centre (-288.1465, 193.0085) radius 2
  circle A10 centre (-198.233, 101.9654) radius 2
  circle A11 centre (-288.1649, 10.9605) radius 2
  point P0 (-382.7081, 102.0177)
  dimension "d113" = 4
  dimension "d114" = 4
  dimension "d115" = 4
  dimension "d116" = 4
  constraint concentric A0 A1
  constraint concentric A4 A5
  constraint concentric A2 A6
  constraint concentric A3 A7
  constraint symmetric A1 L0 A11
  constraint symmetric A4.centre L0 P0
  constraint symmetric A5 L0 A8
  constraint symmetric A6 L0 A9
  constraint symmetric A7 L0 A10
  measures "d113" diameter of A1
  measures "d114" diameter of A5
  measures "d115" diameter of A6
  measures "d116" diameter of A7
extrude "Extrude9" cut sketch "Sketch9" against normal blind 1 contours A1 | A5 | A6 | A7 | A8 | A9 | A10 | A11 bodies 1
split "Split3" by plane through (192.1523, -102.2541, 6.25) normal (-1, 0.000045, 0) bodies 2 1 makes body 4 at (0.8347, -42.7916, 0) makes body 3 at (124.458, -68.6285, 16)
hidden bodies 2 3
equation "d16 = ( 192 * 2 ) * 1 mm"
equation "d87 = ( 192 * 2 ) * 1 mm"
